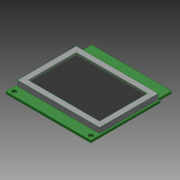
# Autodesk Inventor part: LT24
Saved by Autodesk Inventor 2019.4 (Build 234330000, 330)
## iProperties
Created: 2015-08-09
Part Number: LT24
Material: Phenolharz
Document SubType Name: Modeling
Designer: rYan
Mass: 18.4313 g
Surface Area: 89.6256 cm^2
Volume: 13.356 cm^3
Density: 1.38 g/cm^3
Appearance: Glatt - waldgrün
Author: rYan
Autodesk Inventor part; units mm, degrees
ref_plane "YZ Plane" through (0, 0, 0) normal (1, 0, 0) x (0, 1, 0)
ref_plane "XZ Plane" through (0, 0, 0) normal (0, 1, 0) x (-1, 0, 0)
ref_plane "XY Plane" through (0, 0, 0) normal (0, 0, 1) x (1, 0, 0)
sketch "Skizze1" plane through (0, 0, 0) normal (0, 0, 1) x (1, 0, 0)
  line L0 (-29.2, 4.2) -> (29.2, 4.2)
  line L1 (29.2, 4.2) -> (29.2, -5.8)
  line L2 (29.2, -5.8) -> (31, -5.8)
  line L3 (31, -5.8) -> (31, -56.6)
  line L4 (31, -56.6) -> (-31, -56.6)
  line L5 (-31, -56.6) -> (-31, -5.8)
  line L6 (-31, -5.8) -> (-29.2, -5.8)
  line L7 (-29.2, -5.8) -> (-29.2, 4.2)
  line L8 (-43.4, 0) -> (43.4, 0) projected
  line L9 (0, 16.36) -> (0, -68.76) projected
  point P0 (0, 0)
  dimension "d0" = 4.2
  dimension "d1" = 5.8
  dimension "d2" = 56.6
  dimension "d3" = 62
  dimension "d4" = 58.4
  constraints: 16 end point, 6 perpendicular, 1 horizontal, 1 vertical, 3 other
  measures "d0" distance between parallel lines of L0 L8
  measures "d1" distance between parallel lines of L8 L6
  measures "d2" distance between parallel lines of L4 L8
  measures "d3" distance of L3.end L4.end
  measures "d4" distance of L0.start L0.end
extrude "Extrusion1" add sketch "Skizze1" along normal blind 1.6
sketch "Skizze2" plane through (0, 0, 1.6) normal (0, 0, 1) x (1, 0, 0)
  line L0 (-28, -53.6) -> (28, -53.6) construction
  line L1 (0, 16.36) -> (0, -68.76) construction
  line L2 (-43.4, 0) -> (43.4, 0) construction
  point P0 (0, 0)
  dimension "d7" = 53.6
  dimension "d8" = 56
  constraints: 2 end point, 1 horizontal, 1 symmetric about line
  measures "d7" distance between parallel lines of L0 L2
  measures "d8" distance of L0.start L0.end
hole "Bohrung1" at (-28, -53.6, 1.6) at (28, -53.6, 1.6) direction (0, 0, -1) diameter 3.2 end through all
sketch "Skizze3" plane through (0, 0, 1.6) normal (0, 0, 1) x (1, 0, 0)
  line L0 (0, 16.36) -> (0, -68.76) projected
  line L1 (-43.4, 0) -> (43.4, 0) projected
  line L2 (-30, -6.2) -> (30, -6.2)
  line L3 (30, -6.2) -> (30, -49.2)
  line L4 (30, -49.2) -> (-30, -49.2)
  line L5 (-30, -49.2) -> (-30, -6.2)
  point P0 (0, 0)
  dimension "d16" = 60
  dimension "d17" = 43
  dimension "d18" = 6.2
  constraints: 8 end point, 2 parallel, 1 horizontal, 1 perpendicular, 1 other
  measures "d16" distance of L2.start L2.end
  measures "d17" distance of L4.end L2.start
  measures "d18" distance between parallel lines of L1 L2
extrude "Extrusion2" add sketch "Skizze3" along normal blind 4
shell "Wandung1" thickness 4 removed faces 1 at (10, -20.5333, 5.6)
